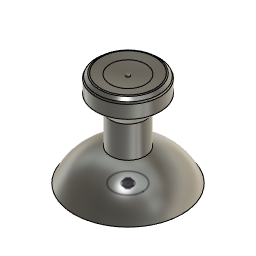
secondary_007mm_thumbstick_loose (Autodesk Fusion 360 design; units mm, degrees)
Autodesk Fusion 360 part; units mm, degrees
other "Base Mesh Feature1"
sketch "Sketch1" plane through (0, 0, 0) normal (0, 0, 1) x (1, 0, 0)
  circle A0 centre (0, 0) radius 1
  circle A1 centre (0, 0) radius 3
  dimension "d1" = 2
  dimension "d8" = 6
  constraint coincident A0.centre A1.centre
  measures "d1" diameter of A0
  measures "d8" diameter of A1
other "Modify1"
other "Modify2"
sketch "Sketch2" plane through (0, 0, 0) normal (0, 1, 0) x (1, 0, 0)
  line L0 (-3.5223, -6.5149) -> (-3.5223, -12.8848)
  line L1 (0.0031, -9.5836) -> (-2.0131, -9.5836)
  line L2 (-3.5223, -12.8848) -> (-6.5394, -15.8715)
  line L3 (-6.5394, -15.8715) -> (-6.5394, -18.506)
  line L4 (-6.3884, -18.8423) -> (-5.7938, -19.3708)
  line L5 (-5.6789, -19.473) -> (-5.6325, -19.4625)
  arc A0 (-5.7938, -19.3708) -> (-5.5297, -19.4395) centre (-5.5945, -19.1466) ccw
  arc A1 (-6.5394, -18.506) -> (-6.3884, -18.8423) centre (-6.0894, -18.506) ccw
  line L6 (-2.0131, -9.5836) -> (-2.0131, -6.8721)
  arc A2 (-2.0131, -6.8721) -> (0, -7.0416) centre (0, 5) ccw
  arc A3 (-10.9545, 0) -> (-3.5223, -6.5149) centre (0, 5) ccw
  arc A4 (-8.6603, 0) -> (0, -5) centre (0, 5) ccw
  line L7 (-10.9545, 0) -> (-8.6603, 0)
  line L8 (0, -7.0416) -> (0, -5)
  arc A5 (-0.3979, -18.9748) -> (0, -19.3623) centre (0, -18.9642) ccw
  line L9 (0, -18.9642) -> (-0.0004, -18.9642)
  line L10 (-0.0004, -18.9642) -> (0, -18.9642)
  line L11 (-5.5297, -19.4395) -> (-3.5918, -19.2064)
  arc A6 (-0.3979, -18.9748) -> (-3.5918, -19.2064) centre (0.4504, -52.8142) ccw
  line L12 (0, -19.3623) -> (0.0031, -9.5836)
  dimension "d4" = 0.3
  dimension "d5" = 0.45
  constraint concentric A2 A4
  constraint horizontal L7
  constraint vertical L6
  constraint vertical L0
  constraint horizontal L1
  constraint tangent L4 A0
  constraint tangent L4 A1
  constraint tangent L3 A1
  constraint concentric A2 A3
  constraint vertical L8
  constraint coincident A5.centre L9.start
  measures "d4" radius of A0
  measures "d5" radius of A1
revolve "Revolve1" add sketch "Sketch2" angle 360 about axis through (0, 0, 19.3623) along (0.000313, 0, -1) makes body 1
sketch "Sketch3" plane through (0, 0, 0) normal (0, 0, 1) x (1, 0, 0)
  line L0 (1.3306, -1.5595) -> (-1.3306, -1.5595)
  line L1 (-20, 0) -> (14, 0) construction
  line L2 (-20, 0) -> (14, 0) construction
  line L3 (1.3306, 1.5595) -> (-1.3306, 1.5595)
  arc A0 (-1.3306, 1.5595) -> (-1.3306, -1.5595) centre (0, 0) ccw
  arc A1 (1.3306, -1.5595) -> (1.3306, 1.5595) centre (0, 0) ccw
  dimension "d9" = 4.1
  constraint coincident A0.centre A1.centre
  constraint horizontal L0
  constraint horizontal L1
  constraint symmetric L2.start L1 L1.start
  constraint symmetric L2.end L1 L1.end
  constraint concentric A0 A1
  measures "d9" diameter of A0
extrude "Extrude1" cut sketch "Sketch3" along normal blind 16 bodies 1
copy_body "Body->Comp1" bodies 1 removing the originals makes body 2 in component "secondary_007mm_thumbstick_loose (1)"
component "secondary_007mm_thumbstick_loose (1)" placed x (1, 0, 0) y (0, 1, 0) z (0, 0, 1) at (0, 0, 0)
named bodies: "secondary_007mm_thumbstick_loose (1)"
